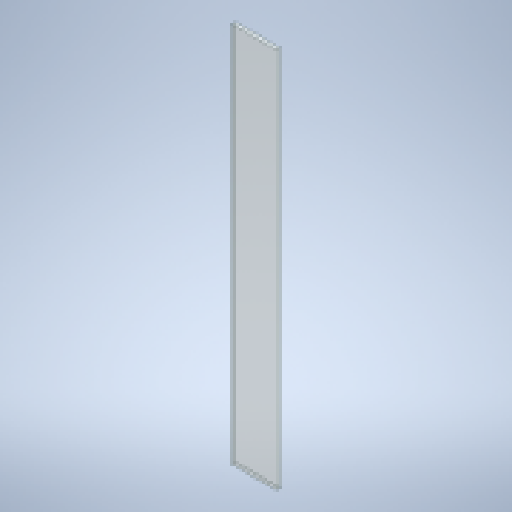
# Autodesk Inventor part: Glasscheibe
Saved by Autodesk Inventor 2025.2 (Build 292293000, 293)
## iProperties
Created: 2025-02-03
Part Number: Glasscheibe
Material: Glas
Document SubType Name: Modeling
Designer: gorenfl4
Mass: 97.3152 g
Surface Area: 250.88 cm^2
Volume: 44.64 cm^3
Density: 2.18 g/cm^3
Appearance: Klar
Author: gorenfl4
Autodesk Inventor part; units mm, degrees
ref_plane "YZ Plane" through (0, 0, 0) normal (1, 0, 0) x (0, 1, 0)
ref_plane "XZ Plane" through (0, 0, 0) normal (0, 1, 0) x (-1, 0, 0)
ref_plane "XY Plane" through (0, 0, 0) normal (0, 0, 1) x (1, 0, 0)
sketch "Skizze1" plane through (0, 0, 0) normal (0, 1, 0) x (-1, 0, 0)
  line L0 (0, 0) -> (-36, 0)
  line L1 (-36, 0) -> (-36, -310)
  line L2 (-36, -310) -> (0, -310)
  line L3 (0, -310) -> (0, 0)
  point P0 (0, 0)
  dimension "d0" = 0
  dimension "d1" = 0
  dimension "d2" = 36
  dimension "d3" = 310
  constraints: 8 end point, 2 parallel, 1 horizontal, 1 perpendicular
  measures "d0" distance from line of L0 point (0, 0)
  measures "d1" distance from line of point (0, 0) L3
  measures "d2" distance between parallel lines of L3 L1
  measures "d3" distance between parallel lines of L2 L0
extrude "Extrusion1" add sketch "Skizze1" along normal blind 3
